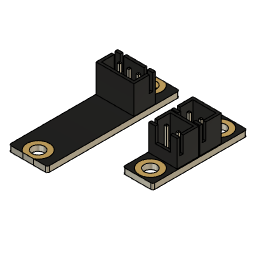
ldo_kirigami_pcbs (Autodesk Fusion 360 design; units mm, degrees)
Autodesk Fusion 360 part; units mm, degrees
note: some values were not read from the file. Chosen so that the rebuilt part matches the saved one: which bodies a step acts on; which face or edge a step refers to.
sketch "Sketch1" plane through (0, 0, 0) normal (0, 0, 1) x (1, 0, 0)
  line L0 (5.5, 5) -> (29.5, 5)
  line L1 (30, 5.5) -> (30, 12.4)
  line L2 (29.5, 12.9) -> (5.5, 12.9)
  line L3 (5, 12.4) -> (5, 5.5)
  line L4 (11.65, 12.9) -> (23.35, 12.9)
  line L5 (23.35, 12.9) -> (23.35, 5)
  line L6 (23.35, 5) -> (11.65, 5)
  line L7 (11.65, 5) -> (11.65, 12.9)
  line L8 (5, 8.95) -> (30, 8.95) construction
  line L9 (8.325, 12.9) -> (8.325, 5) construction
  line L10 (26.675, 12.9) -> (26.675, 5) construction
  circle A0 centre (26.675, 8.95) radius 1.65
  line L11 (11.65, 12.7) -> (17.35, 12.7)
  line L12 (17.35, 12.7) -> (17.35, 5.2)
  line L13 (17.35, 5.2) -> (11.65, 5.2)
  line L14 (11.65, 5.2) -> (11.65, 12.7)
  circle A1 centre (26.675, 8.95) radius 3
  arc A2 (5.5, 12.9) -> (5, 12.4) centre (5.5, 12.4) ccw
  arc A3 (5, 5.5) -> (5.5, 5) centre (5.5, 5.5) ccw
  arc A4 (29.5, 5) -> (30, 5.5) centre (29.5, 5.5) ccw
  arc A5 (30, 12.4) -> (29.5, 12.9) centre (29.5, 12.4) ccw
  line L15 (17.5, 12.9) -> (17.5, 5) construction
  circle A6 centre (8.325, 8.95) radius 1.65
  circle A7 centre (8.325, 8.95) radius 3
  line L16 (23.35, 12.7) -> (17.65, 12.7)
  line L17 (17.65, 12.7) -> (17.65, 5.2)
  line L18 (17.65, 5.2) -> (23.35, 5.2)
  line L19 (23.35, 5.2) -> (23.35, 12.7)
  line L20 (21.15, 7.1) -> (20.55, 7.1)
  line L21 (20.55, 7.1) -> (20.55, 7.7)
  line L22 (20.55, 7.7) -> (21.15, 7.7)
  line L23 (21.15, 7.7) -> (21.15, 7.1)
  line L24 (21.15, 10.8) -> (20.55, 10.8)
  line L25 (21.15, 10.2) -> (21.15, 10.8)
  line L26 (20.55, 10.2) -> (21.15, 10.2)
  line L27 (20.55, 10.8) -> (20.55, 10.2)
  line L28 (15.15, 7.1) -> (14.55, 7.1)
  line L29 (15.15, 7.7) -> (15.15, 7.1)
  line L30 (14.55, 7.7) -> (15.15, 7.7)
  line L31 (14.55, 7.1) -> (14.55, 7.7)
  line L32 (14.55, 10.8) -> (14.55, 10.2)
  line L33 (15.15, 10.8) -> (14.55, 10.8)
  line L34 (15.15, 10.2) -> (15.15, 10.8)
  line L35 (14.55, 10.2) -> (15.15, 10.2)
  line L36 (5.5, -5) -> (39.5, -5)
  line L37 (40, -5.5) -> (40, -14.7)
  line L38 (39.5, -15.2) -> (5.5, -15.2)
  line L39 (5, -14.7) -> (5, -5.5)
  line L40 (11.3, -5.1) -> (17, -5.1)
  line L41 (17, -5.1) -> (17, -15.1)
  line L42 (17, -15.1) -> (11.3, -15.1)
  line L43 (11.3, -15.1) -> (11.3, -5.1)
  line L44 (5, -10.1) -> (40, -10.1) construction
  line L45 (22.5, -5) -> (22.5, -15.2) construction
  line L46 (14.15, -5.1) -> (14.15, -15.1) construction
  line L47 (11.3, -10.1) -> (17, -10.1) construction
  circle A8 centre (37.35, -10.1) radius 1.65
  circle A9 centre (37.35, -10.1) radius 3
  line L48 (39, -7.5) -> (39, -12.5) construction
  arc A10 (40, -5.5) -> (39.5, -5) centre (39.5, -5.5) ccw
  arc A11 (39.5, -15.2) -> (40, -14.7) centre (39.5, -14.7) ccw
  arc A12 (5, -14.7) -> (5.5, -15.2) centre (5.5, -14.7) ccw
  arc A13 (5.5, -5) -> (5, -5.5) centre (5.5, -5.5) ccw
  circle A14 centre (7.65, -10.1) radius 1.65
  circle A15 centre (7.65, -10.1) radius 3
  line L49 (13, -7.3) -> (13.6, -7.3)
  line L50 (13.6, -7.3) -> (13.6, -7.9)
  line L51 (13.6, -7.9) -> (13, -7.9)
  line L52 (13, -7.9) -> (13, -7.3)
  line L53 (13, -9.8) -> (13.6, -9.8)
  line L54 (13, -10.4) -> (13, -9.8)
  line L55 (13.6, -10.4) -> (13, -10.4)
  line L56 (13.6, -9.8) -> (13.6, -10.4)
  line L57 (13, -12.3) -> (13.6, -12.3)
  line L58 (13, -12.9) -> (13, -12.3)
  line L59 (13.6, -12.9) -> (13, -12.9)
  line L60 (13.6, -12.3) -> (13.6, -12.9)
  line L61 (13, -10.1) -> (13.6, -10.1) construction
  line L62 (20, -7.6) -> (25, -7.6)
  line L63 (25, -7.6) -> (25, -12.6)
  line L64 (25, -12.6) -> (20, -12.6)
  line L65 (20, -12.6) -> (20, -7.6)
  line L66 (21.5, -5.8) -> (23.5, -5.8)
  line L67 (23.5, -5.8) -> (23.5, -6.8)
  line L68 (23.5, -6.8) -> (21.5, -6.8)
  line L69 (21.5, -6.8) -> (21.5, -5.8)
  line L70 (23.5, -6.3) -> (21.5, -6.3) construction
  line L71 (22.5, -5.8) -> (22.5, -6.8) construction
  line L72 (21.5, -13.4) -> (21.5, -14.4)
  line L73 (21.5, -14.4) -> (23.5, -14.4)
  line L74 (23.5, -14.4) -> (23.5, -13.4)
  line L75 (23.5, -13.4) -> (21.5, -13.4)
  circle A16 centre (22.5, -10.1) radius 2.25
  line L76 (24.603, -10.9) -> (20.397, -10.9)
  line L77 (24.5156, -11.1) -> (20.4844, -11.1)
  point P0 (30, 5)
  point P1 (30, 12.9)
  point P2 (5, 12.9)
  dimension "d1" = 7.9
  dimension "d2" = 25
  dimension "d4" = 11.7
  dimension "d8" = 3.325
  dimension "d9" = 3.325
  dimension "d10" = 3.3
  dimension "d11" = 7.5
  dimension "d12" = 5.7
  dimension "d13" = 6
  dimension "d14" = 0.5
  dimension "d15" = 0.5
  dimension "d16" = 0.5
  dimension "d36" = 0.6
  dimension "d37" = 0.6
  dimension "d38" = 1.9
  dimension "d41" = 2.2
  dimension "d42" = 0.6
  dimension "d43" = 0.6
  dimension "d44" = 1.9
  dimension "d45" = 2.2
  dimension "d59" = 5
  dimension "d60" = 5
  dimension "d61" = 3.95
  dimension "d63" = 5
  dimension "d64" = 5
  dimension "d65" = 10.2
  dimension "d66" = 35
  dimension "d74" = 12
  dimension "d75" = 5.7
  dimension "d76" = 10
  dimension "d79" = 1
  dimension "d80" = 0.5
  dimension "d81" = 0.5
  dimension "d82" = 0.5
  dimension "d83" = 0.5
  dimension "d84" = 0.5
  dimension "d85" = 5.1
  dimension "d86" = 17.5
  dimension "d88" = 0.6
  dimension "d89" = 0.6
  dimension "d92" = 0
  dimension "d93" = -5
  dimension "d94" = 2.3
  dimension "d95" = 5
  dimension "d96" = 5
  dimension "d97" = 2.6
  dimension "d98" = 15
  dimension "d101" = 2
  dimension "d102" = 1
  dimension "d104" = 1.3
  dimension "d140" = 4.5
  dimension "d144" = 0.2
  dimension "d145" = 1
  constraint horizontal L0
  constraint vertical L1
  constraint horizontal L2
  constraint vertical L3
  constraint horizontal L4
  constraint vertical L5
  constraint horizontal L6
  constraint vertical L7
  constraint coincident L0 L5.end
  constraint coincident L2 L4.start
  constraint coincident L3 L8.start
  constraint coincident L1 L8.end
  constraint perpendicular L1 L8
  constraint coincident L2 L9.start
  constraint coincident L0 L9.end
  constraint perpendicular L0 L9
  constraint coincident L2 L10.start
  constraint coincident L0 L10.end
  constraint perpendicular L0 L10
  constraint midpoint L10 A0.centre
  constraint horizontal L11
  constraint vertical L12
  constraint horizontal L13
  constraint vertical L14
  constraint midpoint L7 L14
  constraint concentric A0 A1
  constraint coincident P2 L2
  constraint coincident P2 L3
  constraint tangent L2 A2
  constraint tangent L3 A2
  constraint coincident L0 L6
  constraint tangent L3 A3
  constraint tangent L0 A3
  constraint equal A2 A3
  constraint coincident P0 L0
  constraint coincident P0 L1
  constraint tangent L0 A4
  constraint tangent L1 A4
  constraint coincident P1 L2
  constraint coincident P1 L1
  constraint tangent L2 A5
  constraint tangent L1 A5
  constraint midpoint L0 L6
  constraint midpoint L4 L15.start
  constraint midpoint L6 L15.end
  constraint symmetric A0 L15 A6
  constraint symmetric A1 L15 A7
  constraint symmetric L11.start L15 L16.start
  constraint symmetric L11.end L15 L16.end
  constraint symmetric L12.end L15 L17.end
  constraint symmetric L13.end L15 L18.end
  constraint horizontal L20
  constraint vertical L21
  constraint horizontal L22
  constraint vertical L23
  constraint symmetric L8 L20.start L24.start
  constraint symmetric L8 L20.end L24.end
  constraint symmetric L8 L21.end L26.start
  constraint symmetric L8 L22.end L25.start
  constraint horizontal L28
  constraint vertical L31
  constraint horizontal L30
  constraint vertical L29
  constraint symmetric L8 L28.end L32.start
  constraint symmetric L8 L28.start L33.start
  constraint symmetric L8 L30.start L32.end
  constraint symmetric L8 L29.start L34.start
  constraint horizontal L36
  constraint vertical L37
  constraint horizontal L38
  constraint vertical L39
  constraint horizontal L40
  constraint vertical L41
  constraint horizontal L42
  constraint vertical L43
  constraint midpoint L40 L46.start
  constraint midpoint L42 L46.end
  constraint midpoint L43 L47.start
  constraint midpoint L41 L47.end
  constraint collinear L44 L47
  constraint coincident L44 A8.centre
  constraint concentric A8 A9
  constraint equal A0 A8
  constraint equal A1 A9
  constraint perpendicular L44 L48
  constraint tangent A8 L48
  constraint coincident L36 L45.start
  constraint coincident L37 L44.end
  constraint tangent L36 A10
  constraint tangent L37 A10
  constraint coincident L38 L45.end
  constraint tangent L37 A11
  constraint tangent L38 A11
  constraint coincident L39 L44.start
  constraint tangent L38 A12
  constraint tangent L39 A12
  constraint tangent L36 A13
  constraint tangent L39 A13
  constraint symmetric L45 A8 A14
  constraint symmetric L45 A9 A15
  constraint horizontal L49
  constraint vertical L50
  constraint horizontal L51
  constraint vertical L52
  constraint midpoint L54 L61.start
  constraint midpoint L56 L61.end
  constraint collinear L44 L61
  constraint horizontal L62
  constraint vertical L63
  constraint horizontal L64
  constraint vertical L65
  constraint horizontal L66
  constraint vertical L67
  constraint horizontal L68
  constraint vertical L69
  constraint midpoint L67 L70.start
  constraint midpoint L69 L70.end
  constraint midpoint L66 L71.start
  constraint midpoint L68 L71.end
  constraint collinear L45 L71
  constraint symmetric L44 L66.start L72.end
  constraint symmetric L44 L66.end L73.end
  constraint symmetric L44 L67.end L74.end
  constraint symmetric L44 L68.end L72.start
  constraint midpoint L45 A16.centre
  constraint coincident A16 L76.start
  constraint coincident A16 L76.end
  constraint perpendicular L45 L76
  constraint coincident A16 L77.start
  constraint coincident A16 L77.end
  constraint perpendicular L45 L77
  measures "d1" distance of P0 P1
  measures "d2" distance of P1 P2
  measures "d4" distance of L5 L7
  measures "d8" distance of L3 L9
  measures "d9" distance of L1 L10
  measures "d10" diameter of A0
  measures "d11" distance of L11 L13
  measures "d12" distance of L12 L14
  measures "d13" diameter of A1
  measures "d14" radius of A2
  measures "d15" radius of A4
  measures "d16" radius of A5
  measures "d36" distance of L20.start L20.end
  measures "d37" distance of L20.start L22.end
  measures "d38" distance of L18 L20
  measures "d41" distance of L19 L23
  measures "d42" distance of L28.end L28.start
  measures "d43" distance of L28.start L29.start
  measures "d44" distance of L13 L28
  measures "d45" distance of L12 L29
  measures "d59" distance of origin L0
  measures "d60" distance of origin L3
  measures "d61" distance of L0 L8
  measures "d63" distance of origin L36
  measures "d64" distance of origin L39
  measures "d65" distance of L36 L38
  measures "d66" distance of L37 L39
  measures "d74" distance of L39 L41
  measures "d75" distance of L41 L43
  measures "d76" distance of L40 L42
  measures "d79" distance of L37 L48
  measures "d80" radius of A10
  measures "d81" radius of A11
  measures "d82" radius of A12
  measures "d83" radius of A13
  measures "d84" radius of A3
  measures "d85" distance of L38 L44
  measures "d86" distance of L39 L45
  measures "d88" distance of L50 L52
  measures "d89" distance of L49 L51
  measures "d94" distance of L43 L60
  measures "d95" distance of L63 L65
  measures "d96" distance of L62 L64
  measures "d97" distance of L38 L64
  measures "d98" distance of L37 L63
  measures "d101" distance of L67 L69
  measures "d102" distance of L66 L68
  measures "d104" distance of L36 L70
  measures "d140" diameter of A16
  measures "d144" distance of L76 L77
  measures "d145" distance of A16.centre L77
extrude "Extrude1" add sketch "Sketch1" along normal blind 1.5 contours L0 L2 L3 L7 L14 A2 A3 | L0 L2 L4 L5 L6 L7 L11 L12 L13 L16 L17 L18 | L0 L1 L2 L5 A4 A5 L19 | L7 L11 L12 L13 L14 | L5 L16 L17 L18 L19 | L20 L21 L22 L23 | L24 L25 L26 L27 | L28 L29 L30 L31 | L32 L33 L34 L35 makes body 1 in component "connector_board"
extrude "Extrude2" add sketch "Sketch1" along normal blind 1.5 separate body contours A1 | A7 makes body 2 at (11.3213, 8.8005, 1) makes body 3 at (29.6713, 8.8005, 1) in component "connector_board"
extrude "Extrude3" add sketch "Sketch1" along normal blind 7 from surface at 1.5 separate body contours L7 L11 L12 L13 L14 | L5 L16 L17 L18 L19 | L20 L21 L22 L23 | L24 L25 L26 L27 | L28 L29 L30 L31 | L32 L33 L34 L35 makes body 4 at (17.65, 10.2, 6.1667) makes body 5 at (17.35, 10.2, 6.1667) in component "connector_board"
copy_body "CutPasteBodies1" bodies 1 2 3 removing the originals makes body 6 makes body 7 makes body 8 in component "connector_pcb"
copy_body "CutPasteBodies1'" bodies 4 5 removing the originals makes body 9 makes body 10 in component "connectors"
shell "Shell1" thickness 0.7 removed faces 2 at (21.45, 7.7, 8.5) at (15.45, 7.7, 8.5) on bodies 9 10 in component "connectors"
sketch "Sketch2" plane through (23.35, 0, 0) normal (1, 0, 0) x (0, 1, 0)
  line L0 (5.2, 1.5) -> (12.7, 1.5)
  line L1 (12.7, 1.5) -> (12.7, 8.75)
  line L2 (12.7, 8.75) -> (5.2, 8.75)
  line L3 (5.2, 8.75) -> (5.2, 1.5)
  line L4 (6.95, 8.75) -> (10.95, 8.75)
  line L5 (10.95, 8.75) -> (10.95, 4.45)
  line L6 (10.95, 4.45) -> (6.95, 4.45)
  line L7 (6.95, 4.45) -> (6.95, 8.75)
  line L8 (5.2, 8.75) -> (12.7, 8.75)
  line L9 (5.2, 1.5) -> (12.7, 1.5)
  line L10 (12.7, 1.5) -> (12.7, 10.5)
  line L11 (12.7, 10.5) -> (5.2, 10.5)
  line L12 (5.2, 10.5) -> (5.2, 1.5)
  line L13 (5.2, 1.5) -> (12.7, 1.5)
  line L14 (12.7, 1.5) -> (12.7, 9)
  line L15 (12.7, 9) -> (5.2, 9)
  line L16 (5.2, 9) -> (5.2, 1.5)
  line L17 (5.2, 1.5) -> (12.7, 1.5)
  line L18 (12.7, 1.5) -> (12.7, 8.5)
  line L19 (12.7, 8.5) -> (5.2, 8.5)
  line L20 (5.2, 8.5) -> (5.2, 1.5)
  dimension "d29" = 4
  dimension "d30" = 4.3
  constraint horizontal L4
  constraint vertical L5
  constraint horizontal L6
  constraint vertical L7
  constraint coincident L2 L4.start
  constraint midpoint L4 L8
  measures "d29" distance of L5 L7
  measures "d30" distance of L4 L6
extrude "Extrude1'" cut sketch "Sketch2" against normal up to surface (0.7 mm away) contours L5 L6 L7 L19 | L2 L4 L5 L7 L8 L19 bodies 9 in component "connectors"
extrude "Extrude2'" cut sketch "Sketch2" along normal up to surface (0.7 mm away) from surface at -6.7 contours L5 L6 L7 L19 | L2 L4 L5 L7 L8 L19 bodies 10 in component "connectors"
extrude "Extrude4" add sketch "Sketch1" along normal blind 7.9 and the other way blind 1.85 separate body contours L20 L21 L22 L23 | L24 L25 L26 L27 | L28 L29 L30 L31 | L32 L33 L34 L35 makes body 11 at (20.75, 7.1, 4.65) makes body 12 at (14.75, 7.1, 4.65) makes body 13 at (20.75, 10.2, 1.4) makes body 14 at (14.95, 10.8, 4.65) in component "connector_board"
chamfer "Chamfer1" distance 0.2 angle 45 8 faces at (14.75, 10.4, -1.85) (14.75, 10.4, 7.9) (20.75, 10.6, -1.85) (20.75, 10.6, 7.9) (20.95, 7.3, -1.85) (20.95, 7.3, 7.9) (14.95, 7.3, -1.85) (14.95, 7.3, 7.9) on bodies 11 12 13 14 in component "connector_board"
copy_body "CutPasteBodies1''" bodies 11 12 13 14 removing the originals makes body 15 makes body 16 makes body 17 makes body 18 in component "pins"
extrude "Extrude5" add sketch "Sketch1" along normal blind 1.5 separate body contours L36 L37 L38 L39 A9 A10 A11 A12 A13 A15 | L40 L41 L42 L43 | L49 L50 L51 L52 | L53 L54 L55 L56 | L57 L58 L59 L60 | L62 L63 L64 L65 | L66 L67 L68 L69 | L72 L73 L74 L75 | A16 L76 | A16 L76 L77 | A16 L77 makes body 19
extrude "Extrude6" add sketch "Sketch1" along normal blind 1.5 separate body contours L39 A15 | L37 A9 picked at (5.3333, -10.1) picked at (39.6667, -10.1) makes body 20 at (5.1508, -11.7595, 1) makes body 21 at (39.8492, -11.7595, 1)
extrude "Extrude7" add sketch "Sketch1" along normal blind 7.5 from surface at 1.5 separate body contours L40 L41 L42 L43 | L49 L50 L51 L52 | L53 L54 L55 L56 | L57 L58 L59 L60 makes body 22
shell "Shell1'" thickness 0.7 removed faces 1 at (13.2, -11.7667, 9) on bodies 22
sketch "Sketch5" plane through (0, 5.9, 0) normal (0, 1, 0) x (-1, 0, 0)
  line L0 (-22.65, 2.2) -> (-18.35, 2.2)
  line L1 (-18.35, 2.2) -> (-18.35, 8.5)
  line L2 (-18.35, 8.5) -> (-22.65, 8.5)
  line L3 (-22.65, 8.5) -> (-22.65, 2.2)
  line L4 (-22.65, 8.5) -> (-21.75, 8.5)
  line L5 (-21.75, 8.5) -> (-21.75, 4.2)
  line L6 (-21.75, 4.2) -> (-22.65, 4.2)
  line L7 (-22.65, 4.2) -> (-22.65, 8.5)
  dimension "d118" = 0.9
  dimension "d119" = 4.3
  constraint horizontal L4
  constraint vertical L5
  constraint horizontal L6
  constraint vertical L7
  constraint coincident L2.end L3.start
  measures "d118" distance of L5 L7
  measures "d119" distance of L4 L6
sketch "Sketch6" plane through (0, 5.9, 0) normal (0, 1, 0) x (-1, 0, 0)
  line L0 (-16.65, 2.2) -> (-12.35, 2.2)
  line L1 (-12.35, 2.2) -> (-12.35, 8.5)
  line L2 (-12.35, 8.5) -> (-16.65, 8.5)
  line L3 (-16.65, 8.5) -> (-16.65, 2.2)
  line L4 (-16.65, 8.5) -> (-15.75, 8.5)
  line L5 (-15.75, 8.5) -> (-15.75, 4.2)
  line L6 (-15.75, 4.2) -> (-16.65, 4.2)
  line L7 (-16.65, 4.2) -> (-16.65, 8.5)
  dimension "d120" = 4.3
  dimension "d121" = 0.9
  constraint horizontal L4
  constraint vertical L5
  constraint horizontal L6
  constraint vertical L7
  constraint coincident L2.end L3.start
  measures "d120" distance of L4 L6
  measures "d121" distance of L5 L7
extrude "Extrude3'" cut sketch "Sketch5" sketch "Sketch6" along normal up to surface and the other way up to surface contours L2 L3 L4 L5 L6 L7 of sketch 2 contours L2 L3 L4 L5 L6 L7 end surface through (17.65, 5.2, 1.5) normal (0, -1, 0) offset 0 second end surface through (11.65, 12.7, 1.5) normal (0, 1, 0) offset 0 bodies 9 10 in component "connectors"
sketch "Sketch1 (2)" plane through (0, 0, 0) normal (0, 1, 0) x (1, 0, 0) in component "neopixel_board"
copy_body "CutPasteBodies1'''" bodies 19 22 20 21 removing the originals makes body 23 makes body 24 makes body 25 makes body 26 in component "neopixel_board"
copy_body "CutPasteBodies1''''" bodies 26 25 23 removing the originals makes body 27 makes body 28 makes body 29 in component "neopixel_pcb"
copy_body "CutPasteBodies1'''''" bodies 24 removing the originals makes body 30 in component "neopixel_connector"
extrude "Extrude1''" add sketch "Sketch1" along normal blind 8.4 and the other way blind 1.85 separate body contours L49 L50 L51 L52 | L53 L54 L55 L56 | L57 L58 L59 L60 makes body 31 at (13.4, -12.3, 4.9833) makes body 32 at (13.4, -9.8, 4.9833) makes body 33 at (13.4, -7.3, 4.9833) in component "neopixel_pcb"
chamfer "Chamfer1'" distance 0.2 angle 45 6 faces at (13.4, -7.7, -1.85) (13.4, -7.7, 8.4) (13.2, -12.5, -1.85) (13.2, -12.5, 8.4) (13.2, -10, -1.85) (13.2, -10, 8.4) on bodies 31 32 33 in component "neopixel_pcb"
extrude "Extrude2''" add sketch "Sketch1" against normal blind 0.5 separate body contours L66 L67 L68 L69 | L72 L73 L74 L75 makes body 34 at (22.1667, -6.1333, 0) makes body 35 at (22.8333, -14.0667, 0) in component "neopixel_pcb"
extrude "Extrude8" add sketch "Sketch1" against normal blind 1.5 separate body contours L62 L63 L64 L65 | A16 L76 | A16 L76 L77 | A16 L77 makes body 36
extrude "Extrude10" cut sketch "Sketch1" along normal blind 0.2 from surface at -1.5 contours A16 L76 | A16 L77 bodies 36
sketch "Sketch8" plane through (0, -14.4, 0) normal (0, 1, 0) x (-1, 0, 0)
  line L0 (-16.3, 2.2) -> (-12, 2.2)
  line L1 (-12, 2.2) -> (-12, 9)
  line L2 (-12, 9) -> (-16.3, 9)
  line L3 (-16.3, 9) -> (-16.3, 2.2)
  line L4 (-12, 9) -> (-12.9, 9)
  line L5 (-12.9, 9) -> (-12.9, 4.7)
  line L6 (-12.9, 4.7) -> (-12, 4.7)
  line L7 (-12, 4.7) -> (-12, 9)
  dimension "d149" = 4.3
  dimension "d150" = 0.9
  constraint horizontal L4
  constraint vertical L5
  constraint horizontal L6
  constraint vertical L7
  constraint coincident L1.end L2.start
  measures "d149" distance of L4 L6
  measures "d150" distance of L5 L7
extrude "Extrude2'''" cut sketch "Sketch8" along normal up to surface (-0.7 mm away) and the other way up to surface (-9.3 mm away) contours L1 L2 L4 L5 L6 L7 bodies 30 in component "neopixel_connector"
sketch "Sketch9" plane through (12, 0, 0) normal (1, 0, 0) x (0, 1, 0)
  line L0 (-14.4, 4.7) -> (-14.4, 2.2)
  line L1 (-14.4, 2.2) -> (-5.8, 2.2)
  line L2 (-5.8, 2.2) -> (-5.8, 4.7)
  line L3 (-5.8, 4.7) -> (-5.1, 4.7)
  line L4 (-5.1, 4.7) -> (-5.1, 9)
  line L5 (-5.1, 9) -> (-15.1, 9)
  line L6 (-15.1, 9) -> (-15.1, 4.7)
  line L7 (-15.1, 4.7) -> (-14.4, 4.7)
  line L8 (-13.7, 9) -> (-12.8, 9)
  line L9 (-12.8, 9) -> (-12.8, 4.7)
  line L10 (-12.8, 4.7) -> (-13.7, 4.7)
  line L11 (-13.7, 4.7) -> (-13.7, 9)
  line L12 (-7.4, 9) -> (-6.5, 9)
  line L13 (-6.5, 9) -> (-6.5, 4.7)
  line L14 (-6.5, 4.7) -> (-7.4, 4.7)
  line L15 (-7.4, 4.7) -> (-7.4, 9)
  dimension "d155" = 1.4
  dimension "d156" = 1.4
  dimension "d157" = 4.3
  dimension "d158" = 4.3
  dimension "d159" = 0.9
  dimension "d160" = 0.9
  constraint horizontal L8
  constraint vertical L9
  constraint horizontal L10
  constraint vertical L11
  constraint coincident L5 L8.start
  constraint horizontal L12
  constraint vertical L13
  constraint horizontal L14
  constraint vertical L15
  constraint coincident L5 L12.start
  measures "d155" distance of L4 L13
  measures "d156" distance of L6 L11
  measures "d157" distance of L8 L10
  measures "d158" distance of L12 L14
  measures "d159" distance of L9 L11
  measures "d160" distance of L13 L15
extrude "Extrude3''" cut sketch "Sketch9" against normal through all contours L5 L8 L9 L10 L11 | L5 L12 L13 L14 L15 bodies 30 in component "neopixel_connector"
copy_body "CutPasteBodies1''''''" bodies 36 removing the originals makes body 37 in component "neopixel_smd"
copy_body "CutPasteBodies2" bodies 34 35 removing the originals makes body 38 makes body 39 in component "neopixel_smd"
component "connector_board" placed x (1, 0, 0) y (0, 1, 0) z (0, 0, 1) at (0, 0, 0)
component "neopixel_board" placed x (1, 0, 0) y (0, 1, 0) z (0, 0, 1) at (0, 0, 0)
component "connector_pcb" placed x (1, 0, 0) y (0, 1, 0) z (0, 0, 1) at (0, 0, 0) in component "connector_board"
component "connectors" placed x (1, 0, 0) y (0, 1, 0) z (0, 0, 1) at (0, 0, 0) in component "connector_board"
component "pins" placed x (1, 0, 0) y (0, 1, 0) z (0, 0, 1) at (0, 0, 0) in component "connectors"
component "neopixel_pcb" placed x (1, 0, 0) y (0, 1, 0) z (0, 0, 1) at (0, 0, 0) in component "neopixel_board"
component "neopixel_connector" placed x (1, 0, 0) y (0, 1, 0) z (0, 0, 1) at (0, 0, 0) in component "neopixel_board"
component "neopixel_smd" placed x (1, 0, 0) y (0, 1, 0) z (0, 0, 1) at (0, 0, 0) in component "neopixel_board"
equation "d1 = connector_pcb_length"
equation "d2 = connector_pcb_width"
equation "d4 = connector_board_contact_width"
equation "connector_pcb_width = 25 mm"
equation "connector_pcb_length = 7.9 mm"
equation "connector_board_contact_width = 11.7 mm"
equation "d8 = ( connector_pcb_width - connector_board_contact_width ) / 2 / 2"
equation "d9 = ( connector_pcb_width - connector_board_contact_width ) / 2 / 2"
equation "d10 = hole_diam"
equation "d11 = connector_length"
equation "d12 = connector_width"
equation "d13 = hole_edge_diam"
equation "d14 = board_radius"
equation "d15 = board_radius"
equation "d16 = board_radius"
equation "board_radius = 0.5 mm"
equation "pcb_thickness = 1.5 mm"
equation "d20 = pcb_thickness"
equation "d22 = pcb_thickness"
equation "d25 = connector_height"
equation "connector_wall = 0.7 mm"
equation "d28 = connector_wall"
equation "d29 = connector_notch_width"
equation "d30 = connector_notch_depth"
equation "d36 = pin_wl"
equation "d37 = pin_wl"
equation "d38 = connector_width / 3"
equation "connector_height = 7 mm"
equation "connector_width = 5.7 mm"
equation "d42 = pin_wl"
equation "d43 = pin_wl"
equation "d44 = connector_width / 3"
equation "d46 = ( connector_height + pcb_thickness ) - 0.6 mm"
equation "neopixel_pcb_width = 10.2 mm"
equation "neopixel_pcb_length = 35 mm"
equation "d65 = neopixel_pcb_width"
equation "d66 = neopixel_pcb_length"
equation "neopixel_connector_width = 10 mm"
equation "neopixel_connector_length = 5.7 mm"
equation "neopixel_connector_height = 7.5 mm"
equation "connector_length = 7.5 mm"
equation "neopixel_connector_from_short_side = 12 mm"
equation "neopixel_led_wl = 5 mm"
equation "neopixel_led_height = 1.5 mm"
equation "d74 = neopixel_connector_from_short_side"
equation "d75 = neopixel_connector_length"
equation "d76 = neopixel_connector_width"
equation "hole_diam = 3.3 mm"
equation "hole_edge_diam = 6 mm"
equation "d80 = board_radius"
equation "d81 = board_radius"
equation "d82 = board_radius"
equation "d83 = board_radius"
equation "d85 = neopixel_pcb_width / 2"
equation "d86 = neopixel_pcb_length / 2"
equation "pin_wl = 0.6 mm"
equation "d88 = pin_wl"
equation "d89 = pin_wl"
equation "d95 = neopixel_led_wl"
equation "d96 = neopixel_led_wl"
equation "d97 = ( neopixel_pcb_width - neopixel_led_wl ) / 2"
equation "d98 = ( neopixel_pcb_length - neopixel_led_wl ) / 2"
equation "smb_l = 2 mm"
equation "smb_w = 1 mm"
equation "d101 = smb_l"
equation "d102 = smb_w"
equation "d104 = ( ( neopixel_pcb_width / 2 ) - ( neopixel_led_wl / 2 ) ) / 2"
equation "pin_chamfer = 0.20 mm"
equation "connector_notch_depth = 4.3 mm"
equation "connector_notch_width = 4 mm"
equation "d108 = pcb_thickness"
equation "d110 = pcb_thickness"
equation "d113 = neopixel_connector_height"
equation "d115 = connector_wall"
equation "d118 = pin_wl * 1.5"
equation "d119 = connector_notch_depth"
equation "d120 = connector_notch_depth"
equation "d121 = pin_wl * 1.5"
equation "d126 = pcb_thickness + neopixel_connector_height - 0.6 mm"
equation "d130 = pcb_thickness + neopixel_connector_height - 0.6 mm"
equation "d134 = pin_chamfer"
equation "smd_h = 0.5 mm"
equation "d136 = -smd_h"
equation "d138 = -neopixel_led_height"
equation "d140 = neopixel_led_wl * 0.9"
equation "d149 = connector_notch_depth"
equation "d150 = pin_wl * 1.5"
equation "d155 = connector_wall * 2"
equation "d156 = connector_wall * 2"
equation "d157 = connector_notch_depth"
equation "d158 = connector_notch_depth"
equation "d159 = pin_wl * 1.5"
equation "d160 = pin_wl * 1.5"
